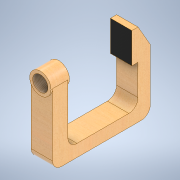
# Autodesk Inventor part: Corpo da Morsa
Saved by Autodesk Inventor 2021 (Build 250183000, 183)
## iProperties
Created: 2021-05-13
Part Number: Corpo da Morsa
Material: Genérico
Document SubType Name: Modeling
Designer: rubia
Density: 1 g/cm^3
Appearance: Pinho amarelo - Sólido claro com pouco brilho
Author: rubia
Autodesk Inventor part; units mm, degrees
ref_plane "YZ Plane" through (0, 0, 0) normal (1, 0, 0) x (0, 1, 0)
ref_plane "XZ Plane" through (0, 0, 0) normal (0, 1, 0) x (-1, 0, 0)
ref_plane "XY Plane" through (0, 0, 0) normal (0, 0, 1) x (1, 0, 0)
sketch "Esboço1" plane through (0, 0, 0) normal (0, 0, 1) x (1, 0, 0)
  circle A0 centre (0, 0) radius 25
  circle A1 centre (0, 0) radius 35
  dimension "d0" = 50
  dimension "d1" = 70
  constraints: 2 centre point, 2 coincident
  measures "d0" diameter of A0
  measures "d1" diameter of A1
extrude "Extrusão1" add sketch "Esboço1" along normal blind 60
sketch "Esboço2" plane through (0, 0, 0) normal (1, 0, 0) x (0, 1, 0)
  line L0 (35, 0) -> (-35, 0) construction
  line L1 (-35, 0) -> (-35, 5) construction
  line L2 (-35, 0) -> (-35, 60) construction
  line L3 (-35, 5) -> (-195, 5)
  line L4 (-35, 60) -> (-35, 55) construction
  line L5 (-35, 55) -> (-235, 55)
  line L6 (-235, 55) -> (-235, -265)
  line L7 (-235, -265) -> (-35, -265)
  line L8 (-35, -265) -> (35, -224.5855)
  line L9 (35, 0) -> (35, -224.5855) construction
  line L10 (35, -224.5855) -> (35, -204.5855)
  line L11 (35, -204.5855) -> (-65, -204.5855)
  line L12 (-65, -204.5855) -> (-65, -224.5855)
  line L13 (-65, -224.5855) -> (-195, -224.5855)
  line L14 (-195, -224.5855) -> (-195, 5)
  line L15 (-35, 55) -> (-35, 5)
  point P0 (0, 0)
  dimension "d4" = 5
  dimension "d5" = 160
  dimension "d6" = 5
  dimension "d7" = 200
  dimension "d8" = 320
  dimension "d9" = 200
  dimension "d10" = 150
  dimension "d11" = 20
  dimension "d12" = 100
  dimension "d13" = 20
  dimension "d14" = 130
  constraints: 28 end point, 5 perpendicular, 4 point on line, 1 collinear, 1 parallel, 1 vertical
  measures "d4" distance of L0.end L1.end
  measures "d5" distance of L1.end L3.end
  measures "d6" distance of L2.end L4.end
  measures "d7" distance of L4.end L5.end
  measures "d8" distance of L5.end L6.end
  measures "d9" distance of L6.end L7.end
  measures "d10" angle of L7 L8
  measures "d11" distance of L8.end L10.end
  measures "d12" distance of L10.end L11.end
  measures "d13" distance of L11.end L12.end
  measures "d14" distance of L12.end L13.end
extrude "Extrusão2" add sketch "Esboço2" along normal mid plane 70
fillet "Arredondamento1" radius 30 4 edges at (0, -235, 55) (0, -195, 5) (0, -235, -265) (0, -195, -224.5855)
sketch "Esboço3" plane through (-35, -35, 5) normal (0, 1, 0) x (1, 0, 0)
  line L0 (70, -20) -> (70, -50) projected
  line L1 (0, 0) -> (70, 0) projected
  line L2 (70, -50) -> (0, -50)
  line L3 (0, -50) -> (0, 0)
  line L4 (0, 0) -> (70, 0)
  line L5 (70, 0) -> (70, -50)
  point P0 (35, 5)
  constraints: 8 end point, 2 parallel, 1 horizontal, 1 perpendicular
extrude "Extrusão3" add sketch "Esboço3" along normal up to next
thread "Rosca1" size "M50x4" class "6H" standard "ANSI Metric M Profile" length 60
